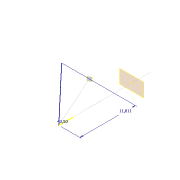
# Autodesk Inventor part: 00_Beampath_v0
Saved by Autodesk Inventor 2022 (Build 260153000, 153)
## iProperties
Created: 2022-04-09
Part Number: 00_Beampath_v0
Material: Generic
Document SubType Name: Modeling
Designer: Prakash Lab
Density: 1 g/cm^3
Appearance: Default
Author: Prakash Lab
Autodesk Inventor part; units mm, degrees
ref_plane "YZ Plane" through (0, 0, 0) normal (1, 0, 0) x (0, 1, 0)
ref_plane "XZ Plane" through (0, 0, 0) normal (0, 1, 0) x (-1, 0, 0)
ref_plane "XY Plane" through (0, 0, 0) normal (0, 0, 1) x (1, 0, 0)
ref_plane "Work Plane1" through (0, 0, 0) normal (0, 0, 1) x (1, 0, 0)
sketch "Sketch1" plane through (0, 0, 0) normal (0, 0, 1) x (1, 0, 0)
  circle A0 centre (0, 0) radius 0.5
  dimension "d0" = 1
  constraints: 1 centre point, 1 coincident
  measures "d0" diameter of A0
extrude "Extrusion1" add sketch "Sketch1" along normal blind 170 and the other way blind 105
sketch "Sketch2" plane through (0, 0, 170) normal (0, 0, 1) x (1, 0, 0)
  circle A0 centre (0, 0) radius 0.5 projected
  circle A1 centre (0, 0) radius 0.8208
  constraints: 1 centre point, 1 coincident
extrude "Extrusion2" add sketch "Sketch2" along normal blind 75 contours A0 | A1
sketch "Sketch3" plane through (0, 0, 245) normal (0, 0, 1) x (1, 0, 0)
  circle A0 centre (0, 0) radius 0.8208 projected
  circle A1 centre (0, 0) radius 0.5 projected
  circle A2 centre (0, 0) radius 0.5
  constraints: 1 centre point, 1 coincident
extrude "Extrusion3" add sketch "Sketch3" along normal blind 75 contours A1
sketch "Sketch4" plane through (0, 0, 320) normal (0, 0, 1) x (1, 0, 0)
  circle A0 centre (0, 0) radius 0.8208 projected
extrude "Extrusion4" add sketch "Sketch4" along normal blind 75
sketch "Sketch5" plane through (0, 0, 0) normal (0, 1, 0) x (-1, 0, 0)
  line L0 (-0.8208, 320) -> (-0.8208, 395) projected
  line L1 (-0.8208, 320) -> (-0.8208, 395) projected
  line L2 (0.8208, 320) -> (0.8208, 395) projected
  line L3 (0.8208, 395) -> (-0.8208, 395) projected
  line L4 (0, 395) -> (201.9828, 145.572)
  point P0 (0, 0)
  dimension "d11" = 39
  dimension "d12" = 249.428
  constraints: 2 end point, 1 midpoint
  measures "d11" angle of L0 L4
  measures "d12" vertical distance of L4.start L4.end
ref_plane "Work Plane2" through (-201.9828, 0, 145.572) normal (-0.6293204, 0, -0.777146) x (0, -1, 0)
sketch "Sketch6" plane through (-201.9828, 0, 145.572) normal (-0.6293204, 0, -0.777146) x (0, -1, 0)
  circle A0 centre (0, 0) radius 0.7121
  point P0 (0, -248.5816)
  constraints: 1 centre point
extrude "Extrusion5" add sketch "Sketch6" against normal up to surface surface through (0, 0, 395) normal (0, 0, 1)
ref_plane "Work Plane3" through (-203.7372, 0.1457, 145.1265) normal (-0.2363825, 0.106463, 0.96581) x (-0.3420657, 0.9212308, -0.1852697)
sketch "Sketch7" plane through (-203.7372, 0.1457, 145.1265) normal (-0.2363825, 0.106463, 0.96581) x (-0.3420657, 0.9212308, -0.1852697)
  point P0 (-42.9382, -158.918)
ref_plane "Work Plane4" through (-201.9828, 0, 145.572) normal (0.2195345, 0.0594809, 0.9737898) x (0.1035983, 0.9910749, -0.0838922)
sketch "Sketch8" plane through (-201.9828, 0, 145.572) normal (0.2195345, 0.0594809, 0.9737898) x (0.1035983, 0.9910749, -0.0838922)
  ellipse E0 centre (0, 0) end of major axis (-0.7121, 0) minor radius 0.6372 projected
  circle A0 centre (0, 0) radius 0.7121
  point P0 (33.1374, -226.717)
  constraints: 1 centre point, 1 coincident, 2 other
extrude "Extrusion6" add sketch "Sketch8" along normal blind 290
body "Solid1"
